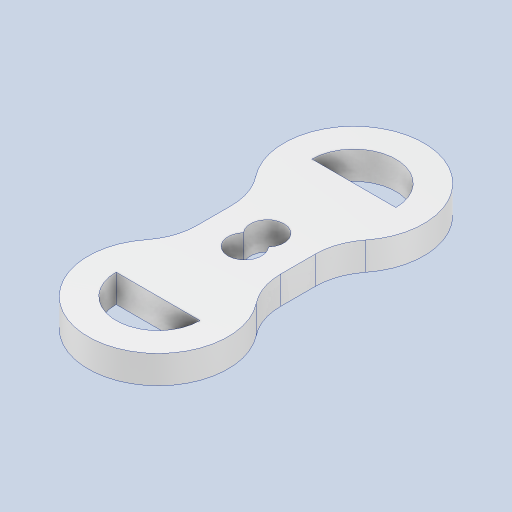
# Autodesk Inventor part: mod5
Saved by Autodesk Inventor 2024 (Build 280153000, 153)
## iProperties
Created: 2025-12-02
Part Number: mod5
Material: Aluminio 6061
Document SubType Name: Modeling
Designer: ANDRES
Density: 2.7 g/cm^3
Appearance: Aluminio - Plano
Author: ANDRES
Autodesk Inventor part; units mm, degrees
ref_plane "YZ Plane" through (0, 0, 0) normal (1, 0, 0) x (0, 1, 0)
ref_plane "XZ Plane" through (0, 0, 0) normal (0, 1, 0) x (-1, 0, 0)
ref_plane "XY Plane" through (0, 0, 0) normal (0, 0, 1) x (1, 0, 0)
sketch "Boceto1" plane through (0, 0, 0) normal (0, 1, 0) x (-1, 0, 0)
  line L0 (0, 35) -> (0, -35) construction
  arc A0 (25, 35) -> (-25, 35) centre (0, 35) ccw
  arc A1 (-25, -35) -> (25, -35) centre (0, -35) ccw
  circle A2 centre (0, -35) radius 15
  circle A3 centre (0, 35) radius 15
  line L1 (0, -20) -> (0, -20)
  line L2 (15, -35) -> (-15, -35)
  line L3 (94.5074, 0) -> (-76.0102, 0) construction
  line L4 (15, 35) -> (-15, 35)
  line L5 (15, -35) -> (-15, -35)
  line L6 (15, -6.1794) -> (-15, -6.1794)
  line L7 (-15, -6.1794) -> (-15, 6.1794)
  line L8 (-15, 6.1794) -> (15, 6.1794)
  line L9 (15, 6.1794) -> (15, -6.1794)
  line L10 (15, -6.1794) -> (-15, 6.1794) construction
  line L11 (-15, -6.1794) -> (15, 6.1794) construction
  circle A4 centre (0, -35) radius 25
  arc A5 (15, -6.1794) -> (19.6273, -19.5155) centre (36.5312, -6.1794) ccw
  line L12 (0, -66.9543) -> (0, 90.1933) construction
  arc A6 (-19.6273, -19.5155) -> (-15, -6.1794) centre (-36.5312, -6.1794) ccw
  circle A7 centre (0, 35) radius 25
  arc A8 (19.6273, 19.5155) -> (15, 6.1794) centre (36.5312, 6.1794) ccw
  arc A9 (-15, 6.1794) -> (-19.6273, 19.5155) centre (-36.5312, 6.1794) ccw
  circle A10 centre (0, 4) radius 6
  circle A11 centre (0, -4) radius 6
  point P0 (0, 0)
  point P1 (0, 60)
  point P2 (0, -60)
  point P3 (0, -20)
  point P4 (15, 35)
  point P5 (0, 0)
  point P6 (15, 6.1794)
  point P7 (25, 35)
  point P8 (-25, 35)
  point P9 (-19.6273, 19.5155)
  point P10 (-15, 6.1794)
  point P11 (-12.5, -0.1825)
  point P12 (-19.6273, -19.5155)
  point P13 (25, -35)
  point P14 (-15, 6.1794)
  point P15 (4.4721, 0)
  point P16 (-4.4721, 0)
  dimension "largo" = 120
  dimension "espesor_junta" = 10
  dimension "d3" = 10
  dimension "d6" = 0
  dimension "d29" = 30
  dimension "d35" = 12
  dimension "d36" = 12
  dimension "d37" = 8
  dimension "d38" = 4
  constraints: 28 end point, 21 point on circle, 12 symmetric about line, 11 centre point, 5 midpoint, 4 horizontal, 4 vertical, 3 coincident, 3 vertical alignment, 2 concentric, 2 parallel, 2 point on line, 2 tangent, 1 perpendicular, 8 other
  measures "largo" distance of point (0, 60) point (0, -60)
  measures "espesor_junta" radial gap between concentric circles of A1 A2
  measures "d3" radial gap between concentric circles of A0 A3
  measures "d6" distance of L1.start L1.end
  measures "d29" distance of L7.end L8.end
  measures "d35" diameter of A10
  measures "d36" diameter of A11
  measures "d37" distance of A10.centre A11.centre
  measures "d38" distance of point (0, 0) A10.centre
extrude "Extrusión8" add sketch "Boceto1" along normal blind 10 contours A7 A0 | A8 L8 A10 A7 | A7 A10 L8 A9 | L9 L6 A11 A10 L8 | L8 A10 A11 L6 L7 | A5 A4 A11 L6 | L6 A11 A4 A6 | A4 A1 | L2 A2 | A3 L4 picked at (1.773, -30.3249) picked at (0.6027, 30.0365)
equation "\"d3\" = espesor_junta"
